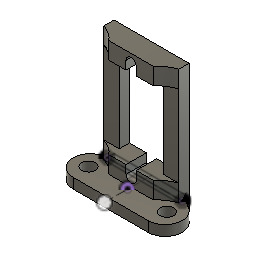
Air Transistor Valve - Motor Holder (Autodesk Fusion 360 design; units mm, degrees)
Autodesk Fusion 360 part; units mm, degrees
note: some values were not read from the file. Chosen so that the rebuilt part matches the saved one: which pieces of a blend or face edit are solid.
sketch "Sketch1" plane through (0, 0, 0) normal (0, 1, 0) x (1, 0, 0)
  line L0 (16, 5) -> (-16, 5)
  line L1 (-16, 5) -> (-16, -5)
  line L2 (-16, -5) -> (16, -5)
  line L3 (16, -5) -> (16, 5)
  line L4 (16, 5) -> (-16, -5) construction
  line L5 (-16, 5) -> (16, -5) construction
  circle A0 centre (-11.5, 0) radius 2
  line L6 (0, 0) -> (0, 15.4432) construction
  circle A1 centre (11.5, 0) radius 2
  dimension "d1" = 32
  dimension "d2" = 10
  dimension "d5" = 23
  dimension "d6" = 4
  constraint horizontal L0
  constraint perpendicular L0 L1
  constraint parallel L0 L2
  constraint parallel L1 L3
  constraint coincident L4 L6.start
  constraint coincident L5 L6.start
  constraint coincident L6.start origin
  constraint perpendicular L0 L6
  constraint symmetric A0 L6 A1
  measures "d1" distance of L0.start L0.end
  measures "d2" distance of L0.start L2.end
  measures "d5" distance of A0.centre A1.centre
  measures "d6" diameter of A0
extrude "Extrude1" add sketch "Sketch1" along normal blind 3 makes body 1
fillet "Fillet1" radius 5 4 edges at (16, 1.5, 5) (16, 1.5, -5) (-16, 1.5, -5) (-16, 1.5, 5) on bodies 1
ref_plane "WorkPlane1" through (0, 3, 0) normal (0, 1, 0) x (1, 0, 0)
sketch "Sketch2" plane through (0, 3, 0) normal (0, 1, 0) x (1, 0, 0)
  line L0 (-11, 7) -> (11, 7)
  line L1 (11, 7) -> (11, 4)
  line L2 (11, 4) -> (-11, 4)
  line L3 (-11, 4) -> (-11, 7)
  line L4 (0, 7) -> (0, -6.8318) construction
  line L5 (11, 5) -> (-11, 5) construction
  line L6 (-11, 5) -> (11, 5)
  dimension "d9" = 2
  dimension "d10" = 22
  dimension "d11" = 1
  constraint horizontal L0
  constraint vertical L1
  constraint horizontal L2
  constraint vertical L3
  constraint midpoint L0 L4.start
  constraint perpendicular L2 L4
  constraint coincident origin L4
  constraint coincident L5.end L6.start
  constraint coincident L5.start L6.end
  measures "d9" distance of L0.end L5
  measures "d10" distance of L0.start L0.end
  measures "d11" distance of L1.end L5.start
extrude "Extrude3" add sketch "Sketch2" along normal blind 34 bodies 1
extrude "Extrude2" add sketch "Sketch2" against normal up to surface (3 mm away) contours L0 L1 L3 L6 bodies 1
fillet "Fillet2" radius 4 2 edges at (11, 1.5, -5) (-11, 1.5, -5) on bodies 1
ref_plane "WorkPlane2" through (0, 20, -4) normal (0, 0, 1) x (1, 0, 0)
sketch "Sketch3" plane through (0, 20, -4) normal (0, 0, 1) x (1, 0, 0)
  line L0 (-6.5, 12) -> (6.5, 12)
  line L1 (6.5, 12) -> (6.5, -12)
  line L2 (6.5, -12) -> (-6.5, -12)
  line L3 (-6.5, -12) -> (-6.5, 12)
  line L4 (11, -17) -> (-11, -17)
  line L5 (0, 12) -> (0, -12) construction
  dimension "d18" = 13
  dimension "d19" = 24
  dimension "d20" = 5
  constraint horizontal L0
  constraint vertical L1
  constraint horizontal L2
  constraint vertical L3
  constraint midpoint L0 L5.start
  constraint midpoint L2 L5.end
  constraint coincident origin L5
  measures "d18" distance of L0.start L0.end
  measures "d19" distance of L0.end L1.end
  measures "d20" distance of L2 L4
extrude "Extrude4" cut sketch "Sketch3" against normal blind 3 bodies 1
ref_plane "WorkPlane3" through (0, 20, -4) normal (0, 0, 1) x (1, 0, 0)
sketch "Sketch4" plane through (0, 20, -4) normal (0, 0, 1) x (1, 0, 0)
  line L0 (-6.5, -12) -> (6.5, -12)
  line L1 (6.5, -12) -> (6.5, -17)
  line L2 (6.5, -17) -> (-6.5, -17)
  line L3 (-6.5, -17) -> (-6.5, -12)
  line L4 (11, -17) -> (-11, -17)
  line L5 (-6.5, 17) -> (6.5, 17)
  line L6 (6.5, 17) -> (6.5, 12)
  line L7 (6.5, 12) -> (-6.5, 12)
  line L8 (-6.5, 12) -> (-6.5, 17)
  line L9 (-11, 17) -> (11, 17)
  point P0 (-6.5, -12)
  point P1 (6.5, -12)
  point P2 (-6.5, 12)
  point P3 (6.5, 12)
  constraint horizontal L0
  constraint vertical L1
  constraint horizontal L2
  constraint vertical L3
  constraint coincident P0 L0.start
  constraint coincident P1 L0.end
  constraint coincident L1.end L4
  constraint horizontal L5
  constraint vertical L6
  constraint horizontal L7
  constraint vertical L8
  constraint coincident P2 L7.end
  constraint coincident P3 L6.end
  constraint coincident L5.end L9
extrude "Extrude5" add sketch "Sketch4" along normal blind 3 bodies 1
ref_plane "WorkPlane4" through (0, 34.5, -1) normal (0, 0, 1) x (1, 0, 0)
sketch "Sketch5" plane through (0, 34.5, -1) normal (0, 0, 1) x (1, 0, 0)
  line L0 (0, 0) -> (0, -38.8634) construction
  line L1 (-6.5, -2.5) -> (6.5, -2.5) construction
  line L2 (-1.5, -2.5) -> (1.5, -2.5)
  line L3 (1.5, -2.5) -> (1.5, 0)
  line L4 (-1.5, 0) -> (-1.5, -2.5)
  arc A0 (1.5, 0) -> (-1.5, 0) centre (0, 0) ccw
  line L5 (-6.5, -2.5) -> (-6.5, -26.5) construction
  line L6 (-6.5, -14.5) -> (19.2348, -14.5) construction
  line L7 (-1.5, -26.5) -> (1.5, -26.5)
  arc A1 (-1.5, -29) -> (1.5, -29) centre (0, -29) ccw
  line L8 (1.5, -26.5) -> (1.5, -29)
  line L9 (-1.5, -29) -> (-1.5, -26.5)
  point P0 (-6.5, -26.5)
  point P1 (0, -29)
  dimension "d27" = 3
  dimension "d28" = 2.5
  constraint vertical L0
  constraint coincident A0.centre L0
  constraint horizontal L2
  constraint vertical L3
  constraint vertical L4
  constraint tangent L4 A0
  constraint tangent L3 A0
  constraint coincident L1 L2.start
  constraint coincident L1.start L5.start
  constraint perpendicular L1 L5
  constraint coincident P0 L5.end
  constraint midpoint L5 L6.start
  constraint perpendicular L5 L6
  constraint symmetric L0.start L6 A1.centre
  constraint symmetric L2.start L6 L7.start
  constraint symmetric L2.end L6 L7.end
  constraint symmetric L3.end L6 A1.end
  constraint symmetric L4.start L6 A1.start
  constraint symmetric A0 L6 A1
  measures "d27" diameter of A0
  measures "d28" distance of L0.start L1
extrude "Extrude6" cut sketch "Sketch5" against normal blind 6 bodies 1
fillet "Fillet3" radius 10 4 edges at (-6.5, 5.5, -4) (-6.5, 34.5, -4) (6.5, 5.5, -4) (6.5, 34.5, -4) on bodies 1
copy_body "Body->Comp1" bodies 1 removing the originals makes body 2 in component "Motor Holder"
component "Motor Holder" placed x (1, 0, 0) y (0, 1, 0) z (0, 0, 1) at (0, 0, 0)
